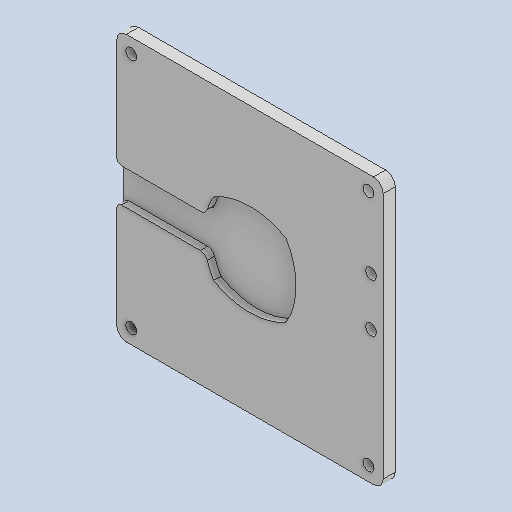
# Autodesk Inventor part: support_camera
Saved by Autodesk Inventor 2024 (Build 280153000, 153)
## iProperties
Created: 2023-03-17
Part Number: support_camera
Material: Generic
Document SubType Name: Modeling
Designer: Thomas
Density: 1 g/cm^3
Appearance: Default
Author: Thomas
Autodesk Inventor part; units mm, degrees
ref_plane "YZ Plane" through (0, 0, 0) normal (1, 0, 0) x (0, 1, 0)
ref_plane "XZ Plane" through (0, 0, 0) normal (0, 1, 0) x (-1, 0, 0)
ref_plane "XY Plane" through (0, 0, 0) normal (0, 0, 1) x (1, 0, 0)
sketch "Sketch1" plane through (0, 0, 0) normal (0, 0, 1) x (1, 0, 0)
  line L0 (-55, -55) -> (55, -55)
  line L1 (55, -55) -> (55, 55)
  line L2 (55, 55) -> (-55, 55)
  line L3 (-55, 55) -> (-55, -55)
  line L4 (-55, -55) -> (55, 55) construction
  line L5 (55, -55) -> (-55, 55) construction
  point P0 (0, 0)
  dimension "d0" = 110
  dimension "d1" = 110
  constraints: 12 end point, 2 midpoint, 2 parallel, 1 horizontal, 1 perpendicular
  measures "d0" distance of L0.end L1.end
  measures "d1" distance of L1.end L2.end
extrude "Extrusion1" add sketch "Sketch1" along normal blind 5
sketch "Sketch2" plane through (0, 0, 5) normal (0, 0, 1) x (1, 0, 0)
  point P0 (0, 0)
  point P1 (-49, 49)
  point P2 (49, 49)
  point P3 (-49, -49)
  point P4 (49, -49)
  dimension "d11" = 98
  dimension "d12" = 98
  dimension "d13" = 49
  dimension "d14" = 49
  constraints: 2 horizontal alignment, 2 vertical alignment
  measures "d11" distance of point (49, 49) point (-49, 49)
  measures "d12" distance of point (-49, -49) point (-49, 49)
  measures "d13" horizontal distance of point (-49, 49) point (0, 0)
  measures "d14" horizontal distance of point (0, 0) point (-49, 49)
hole "Hole1" at (-49, 49, 5) at (49, 49, 5) at (-49, -49, 5) at (49, -49, 5) direction (0, 0, -1) diameter 4.5 depth 8.8 tip angle 118 clearance for "Flat Head Machine Screw" size "M4" standard "Ansi Metric M Profile"
fillet "Fillet1" radius 4 4 edges at (55, 55, 2.5) (55, -55, 2.5) (-55, -55, 2.5) (-55, 55, 2.5)
sketch "Sketch3" plane through (0, 0, 5) normal (0, 0, 1) x (1, 0, 0)
  line L0 (-6.1969, -19) -> (-19, -19)
  line L1 (-19, -19) -> (-19, 19)
  line L2 (-19, 19) -> (19, 19)
  line L3 (19, 19) -> (-6.1969, -19)
  line L4 (-6.1969, -19) -> (-19, 19) construction
  line L5 (-19, -19) -> (19, 19) construction
  line L6 (-55, 51) -> (-55, -51) projected
  arc A0 (-12.2164, 19) -> (-12.2164, -19) centre (11, 0) ccw
  arc A1 (-19, -12.2164) -> (19, -12.2164) centre (0, 11) ccw
  arc A2 (12.2164, -19) -> (12.2164, 19) centre (-11, 0) ccw
  arc A3 (19, 12.2164) -> (-19, 12.2164) centre (0, -11) ccw
  line L7 (-19, -7) -> (-19, 7)
  line L8 (-91.8281, -7) -> (-18.1719, -7)
  line L9 (-18.1719, -7) -> (-18.1719, 7)
  line L10 (-18.1719, 7) -> (-91.8281, 7)
  line L11 (-91.8281, 7) -> (-91.8281, -7)
  line L12 (-91.8281, -7) -> (-18.1719, 7) construction
  line L13 (-18.1719, -7) -> (-91.8281, 7) construction
  point P0 (0, 0)
  point P1 (0, 0)
  point P2 (-19, 0)
  point P3 (0, -19)
  point P4 (19, 0)
  point P5 (0, 19)
  point P6 (-15.2369, 15.7631)
  point P7 (-14.9878, 14.9878)
  point P8 (-46.7631, -15.7631)
  point P9 (14.9878, -14.9878)
  point P10 (-14.9878, -14.9878)
  point P11 (14.9878, 14.9878)
  point P12 (-55, 0)
  point P13 (-55, 7)
  point P14 (-55, -7)
  point P15 (-18.1719, -7)
  dimension "d18" = 38
  dimension "d19" = 38
  dimension "d20" = 30
  dimension "d23" = 360
  dimension "d28" = 42.3919
  dimension "d30" = 14
  constraints: 26 end point, 14 point on circle, 5 midpoint, 4 centre point, 3 parallel, 3 point on line, 2 coincident, 2 horizontal, 2 perpendicular, 1 vertical alignment, 21 other
  measures "d18" distance of L1.end L2.end
  measures "d19" distance between parallel lines of L0 L2
  measures "d20" radius of A0
  measures "d28" distance of point (14.988, 14.988) point (-14.988, -14.988)
  measures "d30" distance of L10.end L8.start
extrude "Extrusion2" cut sketch "Sketch3" against normal blind 3 contours A1 A0 L9 A3 A2 L3 | L3 A2 A1 | L8 L1 A0 | A0 L9 | L8 L6 L10 L1 | L1 L10 A0
fillet "Fillet2" radius 3 4 edges at (14.9878, -14.9878, 3.5) (-14.9878, 14.9878, 3.5) (-18.1719, -7, 3.5) (-18.1719, 7, 3.5)
sketch "Sketch4" plane through (0, 0, 5) normal (0, 0, 1) x (1, 0, 0)
  line L0 (55, -51) -> (55, 51) construction
  line L1 (50, 20) -> (50, 0) construction
  point P0 (0, 0)
  point P1 (55, 0)
  point P2 (50, 10)
  dimension "d40" = 20
  dimension "d43" = 10
  dimension "d44" = 5
  constraints: 2 end point, 2 midpoint, 1 vertical, 1 vertical alignment
  measures "d40" distance of L1.end L1.start
  measures "d43" vertical distance of point (55, 0) point (50, 10)
  measures "d44" distance between parallel lines of L0 L1
hole "Hole2" at (50, 20, 5) at (50, 0, 5) direction (0, 0, -1) diameter 4.5 depth 14.2 tip angle 118 clearance for "Countersunk Flat Head Screw ISO 2009/7046" size "M4" standard "ISO"
fillet "Fillet3" radius 2 2 edges at (-55, -7, 3.5) (-55, 7, 3.5)
equation "\"d0\" = pcb_size"
equation "\"d1\" = pcb_size"
equation "\"d11\" = pcb_fixation_ecart"
equation "\"d12\" = d11"
equation "\"d13\" = 0.5 * d12"
equation "\"d14\" = 0.5 * d11"
equation "\"pcb_size\" = 110"
equation "\"pcb_fixation_ecart\" = 98"
body "Solid1"
